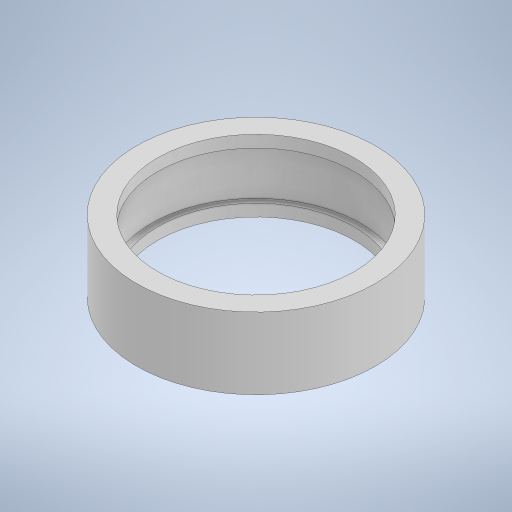
# Autodesk Inventor part: Out
Saved by Autodesk Inventor 2023 (Build 270158000, 158)
## iProperties
Created: 2023-10-09
Part Number: Out
Material: Generic
Document SubType Name: Modeling
Designer: huy20
Density: 1 g/cm^3
Appearance: Default
Author: huy20
Autodesk Inventor part; units mm, degrees
ref_plane "YZ Plane" through (0, 0, 0) normal (1, 0, 0) x (0, 1, 0)
ref_plane "XZ Plane" through (0, 0, 0) normal (0, 1, 0) x (-1, 0, 0)
ref_plane "XY Plane" through (0, 0, 0) normal (0, 0, 1) x (1, 0, 0)
sketch "Sketch1" plane through (0, 0, 0) normal (0, 0, 1) x (1, 0, 0)
  line L0 (-1.5068, 0) -> (-1.5068, 9.9919)
  line L1 (2.6182, 5.5444) -> (2.6182, 6.0444)
  line L2 (2.6182, 6.0444) -> (3.4932, 6.0444)
  line L3 (3.4932, 6.0444) -> (3.4932, 3.0444)
  line L4 (3.4932, 3.0444) -> (2.6182, 3.0444)
  line L5 (2.6182, 3.0444) -> (2.6182, 3.5444)
  line L6 (2.6182, 5.5444) -> (2.8682, 5.5444)
  line L7 (2.8682, 5.5444) -> (2.8682, 3.5444)
  line L8 (2.8682, 3.5444) -> (2.6182, 3.5444)
  dimension "d5" = 3
  dimension "d13" = 0.25
  dimension "d14" = 10
  dimension "d15" = 0.5
  dimension "d16" = 8.75
  constraints: 18 end point, 5 perpendicular, 2 point on line, 2 vertical, 1 collinear, 1 horizontal
  measures "d5" distance of L2.end L3.end
  measures "d13" distance of L1.start L6.end
  measures "d14" diameter of L3 L0
  measures "d15" distance of L1.start L1.end
  measures "d16" diameter of L7 L0
revolve "Revolution1" add sketch "Sketch1" angle 360 about axis through (-1.5068, 0, 0) along (0, 1, 0)
body "Solid1"
